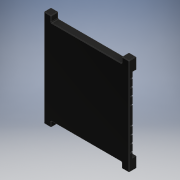
# Autodesk Inventor part: +Y
Saved by Autodesk Inventor 2018 (Build 220112000, 112)
## iProperties
Created: 2018-07-04
Part Number: +Y
Material: Aluminum 6061
Document SubType Name: Modeling
Designer: Bradley
Density: 2.7 g/cm^3
Appearance: Anodized - Dark Gray
Author: Bradley
Autodesk Inventor part; units mm, degrees
ref_plane "YZ Plane" through (0, 0, 0) normal (1, 0, 0) x (0, 1, 0)
ref_plane "XZ Plane" through (0, 0, 0) normal (0, 1, 0) x (-1, 0, 0)
ref_plane "XY Plane" through (0, 0, 0) normal (0, 0, 1) x (1, 0, 0)
sketch "Sketch1" plane through (0, 0, 0) normal (0, 1, 0) x (-1, 0, 0)
  line L0 (50, 57) -> (50, -56.5)
  line L1 (50, -56.5) -> (41.5, -56.5)
  line L2 (41.5, -56.5) -> (41.5, -50)
  line L3 (41.5, -50) -> (-41.5, -50)
  line L4 (-41.5, -50) -> (-41.5, -56.5)
  line L5 (-41.5, -56.5) -> (-50, -56.5)
  line L6 (-50, -56.5) -> (-50, 57)
  line L7 (-50, 57) -> (-41.5, 57)
  line L8 (-41.5, 57) -> (-41.5, 50)
  line L9 (-41.5, 50) -> (41.5, 50)
  line L10 (41.5, 50) -> (41.5, 57)
  line L11 (50, 57) -> (41.5, 57)
  point P0 (0, 0)
  point P1 (0, 50)
  dimension "d0" = 100
  dimension "d1" = 8.5
  dimension "d2" = 113.5
  dimension "d3" = 7
  dimension "d4" = 6.5
  dimension "d5" = 56.5
  constraints: 24 end point, 8 perpendicular, 7 point on line, 1 collinear, 1 midpoint, 1 vertical, 1 vertical alignment
  measures "d0" distance between parallel lines of L6 L0
  measures "d1" distance of L0.start L10.end
  measures "d2" distance of L0.start L0.end
  measures "d3" distance of L9.end L10.end
  measures "d4" distance of L1.end L2.end
  measures "d5" distance from line of point (0, 0) L1
extrude "Extrusion1" add sketch "Sketch1" along normal mid plane 8.5
sketch "Sketch2" plane through (50, -4.25, -56.5) normal (1, 0, 0) x (0, 0, -1)
  line L0 (0, 8.5) -> (0, 0) projected
  line L1 (-113.5, 8.5) -> (0, 8.5) projected
  line L2 (-113.5, 8.5) -> (-113.5, 0) projected
  line L3 (0, 0) -> (-113.5, 0) projected
  line L4 (0, 8.5) -> (-113.5, 8.5) projected
  line L5 (-100.5, 8.5) -> (-100.5, 4)
  line L6 (-100.5, 4) -> (-12.5, 4)
  line L7 (-12.5, 4) -> (-12.5, 8.5)
  line L8 (-46.6, 4) -> (-45.4, 4)
  line L9 (-45.4, 4) -> (-45.4, 2)
  line L10 (-45.4, 2) -> (-46.6, 2)
  line L11 (-46.6, 2) -> (-46.6, 4)
  line L12 (-113.5, 0) -> (0, 0) construction
  line L13 (-56.5, 0) -> (-56.5, 8.5) construction
  line L14 (-37.6, 2) -> (-37.6, 4)
  line L15 (-37.6, 4) -> (-36.4, 4)
  line L16 (-36.4, 2) -> (-37.6, 2)
  line L17 (-36.4, 4) -> (-36.4, 2)
  line L18 (-28.6, 2) -> (-28.6, 4)
  line L19 (-28.6, 4) -> (-27.4, 4)
  line L20 (-27.4, 2) -> (-28.6, 2)
  line L21 (-27.4, 4) -> (-27.4, 2)
  line L22 (-19.6, 2) -> (-19.6, 4)
  line L23 (-19.6, 4) -> (-18.4, 4)
  line L24 (-18.4, 2) -> (-19.6, 2)
  line L25 (-18.4, 4) -> (-18.4, 2)
  line L26 (-66.4, 4) -> (-67.6, 4)
  line L27 (-67.6, 4) -> (-67.6, 2)
  line L28 (-67.6, 2) -> (-66.4, 2)
  line L29 (-66.4, 2) -> (-66.4, 4)
  line L30 (-75.4, 2) -> (-75.4, 4)
  line L31 (-75.4, 4) -> (-76.6, 4)
  line L32 (-76.6, 2) -> (-75.4, 2)
  line L33 (-76.6, 4) -> (-76.6, 2)
  line L34 (-84.4, 2) -> (-84.4, 4)
  line L35 (-84.4, 4) -> (-85.6, 4)
  line L36 (-85.6, 2) -> (-84.4, 2)
  line L37 (-85.6, 4) -> (-85.6, 2)
  line L38 (-93.4, 2) -> (-93.4, 4)
  line L39 (-93.4, 4) -> (-94.6, 4)
  line L40 (-94.6, 2) -> (-93.4, 2)
  line L41 (-94.6, 4) -> (-94.6, 2)
  line L42 (-106.5, 8.5) -> (-106.5, 0) projected
  line L43 (-6.5, 8.5) -> (-6.5, 0) projected
  point P0 (-56.5, 4.25)
  point P1 (-46, 2)
  point P2 (-37, 2)
  point P3 (-28, 2)
  point P4 (-19, 2)
  point P5 (-67, 2)
  point P6 (-76, 2)
  point P7 (-85, 2)
  point P8 (-94, 2)
  dimension "d8" = 4
  dimension "d11" = 1.2
  dimension "d12" = 2
  dimension "d15" = 9
  dimension "d20" = 21
  dimension "d23" = 6
  dimension "d24" = 6
  constraints: 72 end point, 20 symmetric about line, 5 point on line, 4 perpendicular, 2 horizontal, 2 midpoint, 2 parallel, 1 vertical, 27 other
  measures "d8" distance between parallel lines of L6 L3
  measures "d11" distance of L9.end L10.end
  measures "d12" distance between parallel lines of L10 L3
  measures "d15" distance of L8.start L14.end
  measures "d20" distance of point (-46, 2) point (-67, 2)
  measures "d23" distance between parallel lines of L43 L7
  measures "d24" distance between parallel lines of L5 L42
extrude "Extrusion2" cut sketch "Sketch2" against normal through all contours L7 L6 L5 L1 | L25 L24 L22 L6 | L6 L38 L40 L41 | L21 L20 L18 L6 | L6 L34 L36 L37 | L17 L16 L14 L6 | L6 L30 L32 L33 | L9 L10 L11 L6 | L6 L29 L28 L27
fillet "Fillet1" radius 1 6 edges at (41.5, 0, 50) (-41.5, 0, 50) (-41.5, 0, -50) (41.5, 0, -50) (50, -4.25, 0.25) (-50, -4.25, 0.25)
chamfer "Chamfer1" distance 0.5 angle 45 40 edges at (-45.25, -4.25, 57) (-49.7071, -3.9571, 57) (-50, 0.5, 57) (-45.75, 4.25, 57) (-41.5, 0, 57) (0, -4.25, 50) (-41.2071, -4.25, 50.2929) (-41.5, -4.25, 54) (41.2071, -4.25, 50.2929) (41.5, -4.25, 54) (0, 4.25, 50) (41.2071, 4.25, 50.2929) (41.5, 4.25, 54) (-41.2071, 4.25, 50.2929) (-41.5, 4.25, 54) (41.5, 0, 57) (45.25, -4.25, 57) (49.7071, -3.9571, 57) (50, 0.5, 57) (45.75, 4.25, 57) (45.25, -4.25, -56.5) (49.7071, -3.9571, -56.5) (50, 0.5, -56.5) (45.75, 4.25, -56.5) (41.5, 0, -56.5) (41.5, 4.25, -53.75) (41.2071, 4.25, -50.2929) (0, 4.25, -50) (-41.2071, 4.25, -50.2929) (-41.5, 4.25, -53.75) (41.5, -4.25, -53.75) (41.2071, -4.25, -50.2929) (0, -4.25, -50) (-41.2071, -4.25, -50.2929) (-41.5, -4.25, -53.75) (-45.75, 4.25, -56.5) (-50, 0.5, -56.5) (-49.7071, -3.9571, -56.5) (-45.25, -4.25, -56.5) (-41.5, 0, -56.5)
equation "\"d23\" = d24"
body "Solid1"
